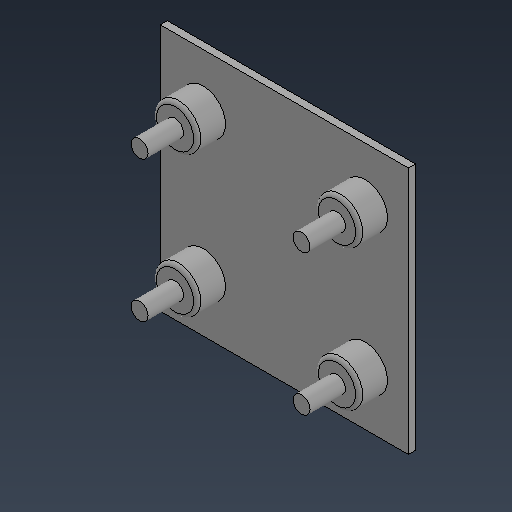
# Autodesk Inventor part: Plateo
Saved by Autodesk Inventor 2026.2 (Build 302298010, 298A)
## iProperties
Created: 2026-06-05
Part Number: Plateo
Material: Generic
Document SubType Name: Modeling
Designer: szymo
Density: 1 g/cm^3
Appearance: Default(1)
Author: szymo
Autodesk Inventor part; units mm, degrees
ref_plane "YZ Plane" through (0, 0, 0) normal (1, 0, 0) x (0, 1, 0)
ref_plane "XZ Plane" through (0, 0, 0) normal (0, 1, 0) x (-1, 0, 0)
ref_plane "Work Plane1" through (0, 0, 3.85) normal (0, 0, 1) x (1, 0, 0)
sketch "Sketch1" plane through (0, 0, 3.85) normal (0, 0, 1) x (1, 0, 0)
  line L0 (-150, -25) -> (-80, -25)
  line L1 (-80, -25) -> (-80, 45)
  line L2 (-80, 45) -> (-150, 45)
  line L3 (-150, 45) -> (-150, -25)
  circle A0 centre (-10, 10) radius 2.5 projected
  line L4 (-150, 0) -> (-150, 5.1) projected
  line L5 (-150, 14.9) -> (-150, 20) projected
  point P0 (0, 0)
  dimension "d0" = 70
  dimension "d20" = 70
  dimension "d21" = 0
  constraints: 8 end point, 2 horizontal, 2 parallel, 1 perpendicular
  measures "d0" distance between parallel lines of L1 L3
  measures "d20" distance of L0.end L1.end
  measures "d21" distance between parallel lines of L3 L4
extrude "Extrusion1" add sketch "Sketch1" along normal blind 2 contours L3 L2 L1 L0
sketch "Sketch2" plane through (0, 0, 5.85) normal (0, 0, 1) x (1, 0, 0)
  line L0 (-80, -25) -> (-80, 45) projected
  line L1 (-80, 45) -> (-150, 45) projected
  line L2 (-150, 45) -> (-150, -25) projected
  line L3 (-150, -25) -> (-80, -25) projected
  circle A0 centre (-137.85, -9.85) radius 2.4
  circle A1 centre (-137.85, 29.85) radius 2.4
  circle A2 centre (-92.15, -9.85) radius 2.4
  circle A3 centre (-92.15, 29.85) radius 2.4
  line L4 (-140.25, -12.25) -> (-89.75, -12.25)
  line L5 (-89.75, -12.25) -> (-89.75, 32.25)
  line L6 (-89.75, 32.25) -> (-140.25, 32.25)
  line L7 (-140.25, 32.25) -> (-140.25, -12.25)
  line L8 (-150, -25) -> (-80, 45) construction
  line L9 (-80, -25) -> (-150, 45) construction
  line L10 (-89.75, -12.25) -> (-140.25, 32.25) construction
  line L11 (-140.25, -12.25) -> (-89.75, 32.25) construction
  point P0 (0, 0)
  point P1 (-115, 10)
  dimension "d5" = 4.8
  dimension "d6" = 4.8
  dimension "d7" = 4.8
  dimension "d8" = 4.8
  dimension "d9" = 44.5
  dimension "d10" = 50.5
  constraints: 16 end point, 8 tangent, 4 centre point, 2 midpoint, 2 parallel, 2 perpendicular, 1 horizontal
  measures "d5" diameter of A0
  measures "d6" diameter of A1
  measures "d7" diameter of A2
  measures "d8" diameter of A3
  measures "d9" distance of L6.end L4.start
  measures "d10" distance between parallel lines of L5 L7
extrude "Extrusion2" add sketch "Sketch2" along normal blind 18 contours A0 | A1 | A2 | A3
sketch "Sketch3" plane through (0, 0, 5.85) normal (0, 0, 1) x (1, 0, 0)
  circle A0 centre (-92.15, -9.85) radius 2.4 projected
  circle A1 centre (-92.15, 29.85) radius 2.4 projected
  circle A2 centre (-137.85, -9.85) radius 2.4 projected
  circle A3 centre (-137.85, 29.85) radius 2.4 projected
  circle A4 centre (-137.85, -9.85) radius 6.25
  circle A5 centre (-137.85, 29.85) radius 6.25
  circle A6 centre (-92.15, -9.85) radius 6.25
  circle A7 centre (-92.15, 29.85) radius 6.25
  point P0 (0, 0)
  dimension "d13" = 12.5
  dimension "d14" = 12.5
  dimension "d15" = 12.5
  dimension "d16" = 12.5
  constraints: 4 centre point, 4 coincident
  measures "d13" diameter of A4
  measures "d14" diameter of A5
  measures "d15" diameter of A6
  measures "d16" diameter of A7
extrude "Extrusion3" add sketch "Sketch3" along normal blind 8
fillet "Fillet1" radius 1 4 edges at (-144.1, -9.85, 13.85) (-98.4, -9.85, 13.85) (-98.4, 29.85, 13.85) (-144.1, 29.85, 13.85)
equation "\"d20\" = d0"
equation "\"d14\" = d13"
equation "\"d15\" = d13"
equation "\"d16\" = d13"
body "Solid1"
